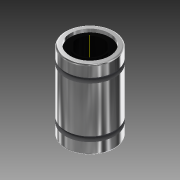
# Autodesk Inventor part: lineair bearing 8 x15 x 24
Saved by Autodesk Inventor 2013 (Build 170138000, 138)
## iProperties
Created: 2012-11-04
Part Number: lineair bearing 8 x15 x 24
Material: Generic
Document SubType Name: Modeling
Designer: Nico
Density: 1 g/cm^3
Author: Nico
Autodesk Inventor part; units mm, degrees
ref_plane "YZ Plane" through (0, 0, 0) normal (1, 0, 0) x (0, 1, 0)
ref_plane "XZ Plane" through (0, 0, 0) normal (0, 1, 0) x (-1, 0, 0)
ref_plane "XY Plane" through (0, 0, 0) normal (0, 0, 1) x (1, 0, 0)
sketch "Sketch1" plane through (0, 0, 0) normal (0, 0, 1) x (1, 0, 0)
  circle A0 centre (0, 0) radius 4
  circle A1 centre (0, 0) radius 6
  dimension "d0" = 8
  dimension "d2" = 12
  constraints: 2 centre point, 2 coincident
  measures "d0" diameter of A0
  measures "d2" diameter of A1
sketch "Sketch1 outline for Extrusion1" plane through (0, 0, 0) normal (0, 0, 1) x (1, 0, 0)
  circle A0 centre (0, 0) radius 6
  circle A1 centre (0, 0) radius 4
extrude "Extrusion1" add sketch "Sketch1 outline for Extrusion1" along normal blind 22
sketch "Sketch2" plane through (0, 0, 22) normal (0, 0, 1) x (1, 0, 0)
  circle A0 centre (0, 0) radius 6 projected
  circle A1 centre (0, 0) radius 7.5
  dimension "d5" = 15
  constraints: 1 centre point, 1 coincident
  measures "d5" diameter of A1
sketch "Sketch2 outline for Extrusion2" plane through (0, 0, 22) normal (0, 0, 1) x (1, 0, 0)
  circle A0 centre (0, 0) radius 7.5
  circle A1 centre (0, 0) radius 6
extrude "Extrusion2" add sketch "Sketch2 outline for Extrusion2" along normal blind 1 and the other way blind 2.5
sketch "Sketch3" plane through (0, 0, 19.5) normal (0, 0, -1) x (-1, 0, 0)
  circle A0 centre (0, 0) radius 6 projected
  circle A1 centre (0, 0) radius 7.5 projected
  circle A2 centre (0, 0) radius 7
  dimension "d11" = 14
  constraints: 1 centre point, 1 coincident
  measures "d11" diameter of A2
sketch "Sketch3 outline for Extrusion3" plane through (0, 0, 19.5) normal (0, 0, -1) x (-1, 0, 0)
  circle A0 centre (0, 0) radius 7
  circle A1 centre (0, 0) radius 6
extrude "Extrusion3" add sketch "Sketch3 outline for Extrusion3" along normal blind 1.5
sketch "Sketch4" plane through (0, 0, 18) normal (0, 0, -1) x (-1, 0, 0)
  circle A0 centre (0, 0) radius 6 projected
  circle A1 centre (0, 0) radius 7 projected
  circle A2 centre (0, 0) radius 7.5
  dimension "d15" = 15
  constraints: 1 centre point, 1 coincident
  measures "d15" diameter of A2
sketch "Sketch4 outline for Extrusion4" plane through (0, 0, 18) normal (0, 0, -1) x (-1, 0, 0)
  circle A0 centre (0, 0) radius 7.5
  circle A1 centre (0, 0) radius 6
extrude "Extrusion4" add sketch "Sketch4 outline for Extrusion4" along normal blind 14
sketch "Sketch5" plane through (0, 0, 4) normal (0, 0, -1) x (-1, 0, 0)
  circle A0 centre (0, 0) radius 6 projected
  circle A1 centre (0, 0) radius 7.5 projected
  circle A2 centre (0, 0) radius 7
  dimension "d19" = 14
  constraints: 1 centre point, 1 coincident
  measures "d19" diameter of A2
sketch "Sketch5 outline for Extrusion5" plane through (0, 0, 4) normal (0, 0, -1) x (-1, 0, 0)
  circle A0 centre (0, 0) radius 7
  circle A1 centre (0, 0) radius 6
extrude "Extrusion5" add sketch "Sketch5 outline for Extrusion5" along normal blind 1.5
sketch "Sketch6" plane through (0, 0, 2.5) normal (0, 0, -1) x (-1, 0, 0)
  circle A0 centre (0, 0) radius 6 projected
  circle A1 centre (0, 0) radius 7 projected
  circle A2 centre (0, 0) radius 7.5
  dimension "d23" = 15
  constraints: 1 centre point, 1 coincident
  measures "d23" diameter of A2
sketch "Sketch6 outline for Extrusion6" plane through (0, 0, 2.5) normal (0, 0, -1) x (-1, 0, 0)
  circle A0 centre (0, 0) radius 7.5
  circle A1 centre (0, 0) radius 6
extrude "Extrusion6" add sketch "Sketch6 outline for Extrusion6" along normal blind 3.5
fillet "Fillet1" radius 1 4 edges at (7, 0, 19.5) (7, 0, 4) (7, 0, 2.5) (7, 0, 18)
fillet "Fillet2" radius 0.5 2 edges at (-7.5, 0, 23) (7.5, 0, -1)
sketch "Sketch7" plane through (0, 0, 22) normal (0, 0, 1) x (1, 0, 0)
  circle A0 centre (0, 0) radius 4 projected
  circle A1 centre (0, 0) radius 6 projected
  circle A2 centre (0, 0) radius 4.5
  dimension "d29" = 9
  constraints: 1 centre point, 1 coincident
  measures "d29" diameter of A2
sketch "Sketch7 outline for Extrusion7" plane through (0, 0, 22) normal (0, 0, 1) x (1, 0, 0)
  circle A0 centre (0, 0) radius 4.5
  circle A1 centre (0, 0) radius 4
extrude "Extrusion7" add sketch "Sketch7 outline for Extrusion7" along normal blind 0.5
sketch "Sketch8" plane through (0, 0, 0) normal (0, 0, -1) x (-1, 0, 0)
  circle A0 centre (0, 0) radius 4 projected
  circle A1 centre (0, 0) radius 6 projected
  circle A2 centre (0, 0) radius 4.5
  dimension "d34" = 9
  constraints: 1 centre point, 1 coincident
  measures "d34" diameter of A2
sketch "Sketch8 outline for Extrusion8" plane through (0, 0, 0) normal (0, 0, -1) x (-1, 0, 0)
  circle A0 centre (0, 0) radius 4.5
  circle A1 centre (0, 0) radius 4
extrude "Extrusion8" add sketch "Sketch8 outline for Extrusion8" along normal blind 0.5
body "Solid1"
